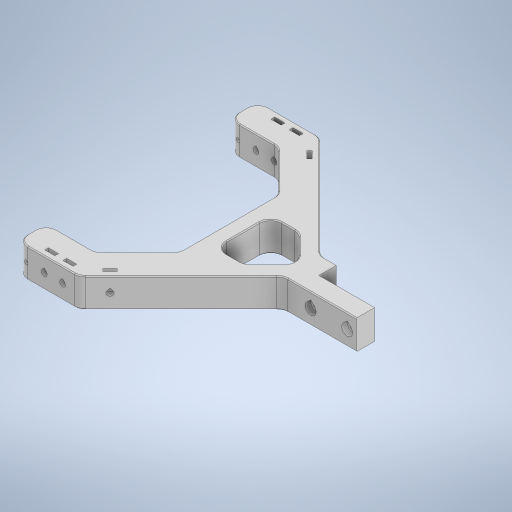
# Autodesk Inventor part: middle_Y
Saved by Autodesk Inventor 2023.1 (Build 271208000, 208)
## iProperties
Created: 2023-11-20
Part Number: middle_Y
Material: Všeobecné
Document SubType Name: Modeling
Designer: zavrel
Density: 1 g/cm^3
Appearance: Výchozí
Author: zavrel
Autodesk Inventor part; units mm, degrees
ref_plane "YZ Plane" through (0, 0, 0) normal (1, 0, 0) x (0, 1, 0)
ref_plane "XZ Plane" through (0, 0, 0) normal (0, 1, 0) x (-1, 0, 0)
ref_plane "XY Plane" through (0, 0, 0) normal (0, 0, 1) x (1, 0, 0)
sketch "Náčrt1" plane through (0, 0, 0) normal (0, 1, 0) x (-1, 0, 0)
  line L0 (0, 0) -> (0, 10)
  line L1 (0, 10) -> (40, 10)
  line L2 (40, 10) -> (96, 66)
  line L3 (96, 66) -> (130, 66)
  line L4 (130, 66) -> (130, 50)
  line L5 (130, 50) -> (102.627417, 50)
  line L6 (102.627417, 50) -> (80, 27.372583)
  line L7 (80, 27.372583) -> (80, 0)
  line L8 (0, 0) -> (258.3801, 0) construction
  line L9 (0, 0) -> (0, -10)
  line L10 (0, -10) -> (40, -10)
  line L11 (40, -10) -> (96, -66)
  line L12 (96, -66) -> (130, -66)
  line L13 (130, -66) -> (130, -50)
  line L14 (130, -50) -> (102.627417, -50)
  line L15 (102.627417, -50) -> (80, -27.372583)
  line L16 (80, -27.372583) -> (80, 0)
  dimension "d0" = 16
  dimension "d2" = 16
  dimension "d3" = 45
  dimension "d4" = 10
  dimension "d5" = 40
  dimension "d7" = 100
  dimension "d9" = 80
  dimension "d10" = 50
  constraints: 34 end point, 7 symmetric about line, 3 perpendicular, 2 horizontal, 2 parallel, 1 point on line, 1 vertical
  measures "d0" distance of L3.end L4.end
  measures "d2" distance between parallel lines of L6 L2
  measures "d3" angle of L8 L2
  measures "d4" distance between parallel lines of L8 L1
  measures "d5" distance of L9.end L10.end
  measures "d7" distance between parallel lines of L14 L5
  measures "d9" distance between parallel lines of L9 L16
  measures "d10" distance between parallel lines of L16 L13
extrude "Vysunutí1" add sketch "Náčrt1" along normal blind 16
sketch "Náčrt2" plane through (-96, 0, -66) normal (0, 0, -1) x (-1, 0, 0)
  line L0 (0, 0) -> (34, 0)
  line L1 (34, 0) -> (34, 16)
  line L2 (0, 16) -> (34, 16)
  line L3 (0, 0) -> (0, 16)
  line L4 (34, 8) -> (0, 8) construction
  circle A0 centre (29, 8) radius 1
  circle A1 centre (19, 8) radius 1.6
  circle A2 centre (9, 8) radius 1.6
  line L5 (19, 8) -> (19, 11.827062) construction
  line L6 (19, 10.262742) -> (20.131371, 9.131371)
  line L7 (19, 10.262742) -> (17.868629, 9.131371)
  line L8 (9, 10.262742) -> (10.131371, 9.131371)
  line L9 (9, 10.262742) -> (7.868629, 9.131371)
  point P0 (-96, 0)
  point P1 (7.868629, 9.131371)
  point P2 (10.131371, 9.131371)
  dimension "d13" = 2
  dimension "d14" = 3.2
  dimension "d15" = 5
  dimension "d16" = 10
  dimension "d17" = 10
  dimension "d22" = 90
  dimension "d23" = 90
  constraints: 12 end point, 4 point on line, 3 centre point, 2 midpoint, 2 point on circle, 2 tangent, 1 equal radius, 1 vertical
  measures "d13" diameter of A0
  measures "d14" diameter of A1
  measures "d15" distance from line of L1 A0.centre
  measures "d16" distance of A0.centre L5.start
  measures "d17" distance of L5.start A2.centre
  measures "d22" angle of L7 L6
  measures "d23" angle of L9 L8
extrude "Vysunutí2" cut sketch "Náčrt2" against normal up to surface (132 mm away) contours A0 | A1 | A1 L7 L6 | A2 | A2 L9 L8
sketch "Náčrt3" plane through (-96, 0, -66) normal (0.7071068, 0, -0.7071068) x (-0.7071068, 0, -0.7071068)
  line L0 (-79.195959, 0) -> (0, 0)
  line L1 (0, 0) -> (0, 16)
  line L2 (-79.195959, 16) -> (0, 16)
  line L3 (-79.195959, 0) -> (-79.195959, 16)
  line L4 (0, 8) -> (-20.182521, 8) construction
  circle A0 centre (-12, 8) radius 1.6
  line L5 (-12, 8) -> (-12, 19.241731) construction
  line L6 (-12, 10.262742) -> (-10.868629, 9.131371)
  line L7 (-12, 10.262742) -> (-13.131371, 9.131371)
  point P0 (-114.551299, 0)
  dimension "d20" = 3.2
  dimension "d21" = 90
  dimension "d26" = 12
  constraints: 8 end point, 2 point on circle, 2 point on line, 2 tangent, 1 centre point, 1 horizontal, 1 midpoint, 1 vertical
  measures "d20" diameter of A0
  measures "d21" angle of L7 L6
  measures "d26" distance from line of L1 L5.start
extrude "Vysunutí3" cut sketch "Náčrt3" against normal up to surface (16 mm away) contours A0 | A0 L7 L6
sketch "Náčrt4" plane through (-40, 0, 10) normal (0.7071068, 0, 0.7071068) x (0.7071068, 0, -0.7071068)
  line L0 (-79.195959, 0) -> (0, 0)
  line L1 (0, 0) -> (0, 16)
  line L2 (-79.195959, 16) -> (0, 16)
  line L3 (-79.195959, 0) -> (-79.195959, 16)
  line L4 (-79.195959, 8) -> (0, 8) construction
  circle A0 centre (-67.195959, 8) radius 1.6
  line L5 (-67.195959, 8) -> (-67.195959, 16) construction
  line L6 (-67.195959, 10.262742) -> (-68.32733, 9.131371)
  line L7 (-67.195959, 10.262742) -> (-66.064589, 9.131371)
  point P0 (35.355339, 0)
  dimension "d27" = 3.2
  dimension "d28" = 12
  dimension "d29" = 90
  constraints: 8 end point, 3 point on line, 2 midpoint, 2 point on circle, 2 tangent, 1 centre point, 1 perpendicular
  measures "d27" diameter of A0
  measures "d28" distance from line of L3 L5.start
  measures "d29" angle of L7 L6
extrude "Vysunutí4" cut sketch "Náčrt4" against normal up to surface (16 mm away) contours A0 | A0 L6 L7
sketch "Sketch6" plane through (0, 16, 0) normal (0, 1, 0) x (1, 0, 0)
  line L0 (-130, -66) -> (-96, -66)
  line L1 (-96, -66) -> (-40, -10)
  line L2 (-96, 66) -> (-130, 66)
  line L3 (-40, 10) -> (-96, 66)
  line L4 (-117.75, -63) -> (-112.25, -63)
  line L5 (-112.25, -63) -> (-112.25, -61)
  line L6 (-112.25, -61) -> (-117.75, -61)
  line L7 (-117.75, -61) -> (-117.75, -63)
  line L8 (-117.75, -63) -> (-112.25, -61) construction
  line L9 (-112.25, -63) -> (-117.75, -61) construction
  line L10 (-107.75, -63) -> (-102.25, -63)
  line L11 (-102.25, -63) -> (-102.25, -61)
  line L12 (-102.25, -61) -> (-107.75, -61)
  line L13 (-107.75, -61) -> (-107.75, -63)
  line L14 (-107.75, -63) -> (-102.25, -61) construction
  line L15 (-102.25, -63) -> (-107.75, -61) construction
  line L16 (-87.691495, -53.448855) -> (-91.580583, -57.337942)
  line L17 (-91.580583, -57.337942) -> (-92.994796, -55.923728)
  line L18 (-92.994796, -55.923728) -> (-89.105709, -52.034641)
  line L19 (-89.105709, -52.034641) -> (-87.691495, -53.448855)
  line L20 (-87.691495, -53.448855) -> (-92.994796, -55.923728) construction
  line L21 (-91.580583, -57.337942) -> (-89.105709, -52.034641) construction
  line L22 (-130, -50) -> (-130, -66)
  line L23 (-96, -66) -> (-99.792003, -62.207997) construction
  line L24 (-80, 27.372583) -> (-80, -27.372583)
  line L25 (-80, 0) -> (-94.372603, 0) construction
  line L26 (-117.75, 63) -> (-112.25, 63)
  line L27 (-112.25, 63) -> (-112.25, 61)
  line L28 (-112.25, 61) -> (-117.75, 61)
  line L29 (-117.75, 61) -> (-117.75, 63)
  line L30 (-117.75, 63) -> (-112.25, 61) construction
  line L31 (-112.25, 63) -> (-117.75, 61) construction
  line L32 (-107.75, 63) -> (-102.25, 63)
  line L33 (-102.25, 63) -> (-102.25, 61)
  line L34 (-102.25, 61) -> (-107.75, 61)
  line L35 (-107.75, 61) -> (-107.75, 63)
  line L36 (-107.75, 63) -> (-102.25, 61) construction
  line L37 (-102.25, 63) -> (-107.75, 61) construction
  line L38 (-87.691495, 53.448855) -> (-91.580583, 57.337942)
  line L39 (-91.580583, 57.337942) -> (-92.994796, 55.923728)
  line L40 (-92.994796, 55.923728) -> (-89.105709, 52.034641)
  line L41 (-89.105709, 52.034641) -> (-87.691495, 53.448855)
  line L42 (-87.691495, 53.448855) -> (-92.994796, 55.923728) construction
  line L43 (-91.580583, 57.337942) -> (-89.105709, 52.034641) construction
  point P0 (0, 0)
  point P1 (-115, -62)
  point P2 (-105, -62)
  point P3 (-90.343146, -54.686292)
  point P4 (-115, 62)
  point P5 (-105, 62)
  point P6 (-90.343146, 54.686292)
  dimension "d53" = 2
  dimension "d54" = 5.5
  dimension "d55" = 15
  dimension "d56" = 10
  dimension "d57" = 12
  dimension "d60" = 3
  dimension "d61" = 3
  constraints: 76 end point, 15 symmetric about line, 9 midpoint, 8 parallel, 4 equal length, 3 horizontal, 3 perpendicular, 2 point on line
  measures "d53" distance of L6.end L4.start
  measures "d54" distance of L5.end L6.end
  measures "d55" distance from line of L22 point (-115, -62)
  measures "d56" distance of point (-105, -62) point (-115, -62)
  measures "d57" distance from line of point (-90.343, -54.686) L23
  measures "d60" distance between parallel lines of L1 L16
  measures "d61" distance between parallel lines of L0 L10
extrude "Extrusion5" cut sketch "Sketch6" against normal blind 11
sketch "Sketch7" plane through (0, 0, -10) normal (0, 0, -1) x (-1, 0, 0)
  line L0 (0, 0) -> (40, 0)
  line L1 (40, 0) -> (40, 16)
  line L2 (0, 16) -> (40, 16)
  line L3 (0, 0) -> (0, 16)
  line L4 (0, 8) -> (40, 8) construction
  line L5 (40, 0) -> (40, 16) construction
  circle A0 centre (5, 8) radius 1.6
  circle A1 centre (25, 8) radius 1.6
  line L6 (5, 8) -> (5, 13.898032) construction
  line L7 (5, 10.262742) -> (3.868629, 9.131371)
  line L8 (5, 10.262742) -> (6.131371, 9.131371)
  line L9 (25, 10.262742) -> (23.868629, 9.131371)
  line L10 (25, 10.262742) -> (26.131371, 9.131371)
  dimension "d62" = 3.2
  dimension "d63" = 5
  dimension "d64" = 20
  dimension "d65" = 90
  dimension "d66" = 90
  constraints: 12 end point, 3 point on line, 1 centre point, 1 midpoint, 1 vertical, 7 other
  measures "d63" distance from line of L3 L6.start
  measures "d64" distance of A1.centre L6.start
  measures "d65" angle of L8 L7
  measures "d66" angle of L10 L9
extrude "Extrusion6" cut sketch "Sketch7" against normal through all contours A0 | A0 L7 L8 | A1 | A1 L9 L10
sketch "Sketch8" plane through (0, 0, -10) normal (0, 0, -1) x (-1, 0, 0)
  line L0 (23.868629, 9.131371) -> (25, 10.262742)
  line L1 (25, 10.262742) -> (26.131371, 9.131371)
  arc A0 (23.868629, 9.131371) -> (26.131371, 9.131371) centre (25, 8) ccw
  line L2 (3.868629, 9.131371) -> (5, 10.262742)
  line L3 (5, 10.262742) -> (6.131371, 9.131371)
  arc A1 (3.868629, 9.131371) -> (6.131371, 9.131371) centre (5, 8) ccw
  line L4 (0, 0) -> (40, 0)
  line L5 (40, 0) -> (40, 16)
  line L6 (0, 16) -> (40, 16)
  line L7 (0, 0) -> (0, 16)
  line L8 (40, 16) -> (0, 16)
  line L9 (30.5, 16) -> (30.5, 0)
  line L10 (0, 0) -> (40, 0)
  dimension "d69" = 30.5
  constraints: 2 end point, 2 point on line, 1 perpendicular
  measures "d69" distance between parallel lines of L9 L7
extrude "Extrusion7" cut sketch "Sketch8" against normal blind 10 contours L7 L6 L9 L4
sketch "Sketch9" plane through (0, 16, 0) normal (0, 1, 0) x (1, 0, 0)
  line L0 (-80, 27.372583) -> (-80, -27.372583) construction
  line L1 (-80, 0) -> (-30.631309, 0) construction
  line L2 (-72, 0) -> (-72, -15)
  line L3 (-72, -15) -> (-56.313708, -15)
  line L4 (-56.313708, -15) -> (-41.313708, 0)
  line L5 (0, 0) -> (-30.5, 0)
  line L6 (-30.5, 0) -> (-30.5, 10)
  line L7 (-30.5, 10) -> (-40, 10)
  line L8 (-40, 10) -> (-96, 66)
  line L9 (-96, 66) -> (-130, 66)
  line L10 (-130, 66) -> (-130, 50)
  line L11 (-130, 50) -> (-102.627417, 50)
  line L12 (-102.627417, 50) -> (-80, 27.372583)
  line L13 (-80, 27.372583) -> (-80, -27.372583)
  line L14 (-80, -27.372583) -> (-102.627417, -50)
  line L15 (-102.627417, -50) -> (-130, -50)
  line L16 (-130, -50) -> (-130, -66)
  line L17 (-130, -66) -> (-96, -66)
  line L18 (-96, -66) -> (-40, -10)
  line L19 (-40, -10) -> (0, -10)
  line L20 (0, -10) -> (0, 0)
  line L21 (-112.25, 63) -> (-112.25, 61)
  line L22 (-112.25, 61) -> (-117.75, 61)
  line L23 (-117.75, 61) -> (-117.75, 63)
  line L24 (-117.75, 63) -> (-112.25, 63)
  line L25 (-107.75, -61) -> (-102.25, -61)
  line L26 (-102.25, -61) -> (-102.25, -63)
  line L27 (-102.25, -63) -> (-107.75, -63)
  line L28 (-107.75, -63) -> (-107.75, -61)
  line L29 (-117.75, -61) -> (-112.25, -61)
  line L30 (-112.25, -61) -> (-112.25, -63)
  line L31 (-112.25, -63) -> (-117.75, -63)
  line L32 (-117.75, -63) -> (-117.75, -61)
  line L33 (-107.75, 61) -> (-107.75, 63)
  line L34 (-107.75, 63) -> (-102.25, 63)
  line L35 (-102.25, 63) -> (-102.25, 61)
  line L36 (-102.25, 61) -> (-107.75, 61)
  line L37 (-91.580583, -57.337942) -> (-92.994796, -55.923728)
  line L38 (-92.994796, -55.923728) -> (-89.105709, -52.034641)
  line L39 (-89.105709, -52.034641) -> (-87.691495, -53.448855)
  line L40 (-87.691495, -53.448855) -> (-91.580583, -57.337942)
  line L41 (-87.691495, 53.448855) -> (-89.105709, 52.034641)
  line L42 (-89.105709, 52.034641) -> (-92.994796, 55.923728)
  line L43 (-92.994796, 55.923728) -> (-91.580583, 57.337942)
  line L44 (-91.580583, 57.337942) -> (-87.691495, 53.448855)
  line L45 (-72, 0) -> (-72, 15)
  line L46 (-72, 15) -> (-56.313708, 15)
  line L47 (-56.313708, 15) -> (-41.313708, 0)
  line L48 (-96, -66) -> (-40, -10)
  dimension "d72" = 30
  dimension "d73" = 8
  dimension "d74" = 8
  constraints: 14 end point, 2 point on line, 2 symmetric about line, 1 horizontal, 1 midpoint, 1 parallel, 1 perpendicular, 1 vertical
  measures "d72" distance between parallel lines of L46 L3
  measures "d73" distance between parallel lines of L0 L2
  measures "d74" distance between parallel lines of L18 L4
extrude "Extrusion8" cut sketch "Sketch9" against normal through all contours L45 L46 L47 L4 L3 L2
sketch "Sketch10" plane through (-40, 0, 10) normal (0, 0, 1) x (1, 0, 0)
  line L0 (15, 10.262742) -> (16.131371, 9.131371)
  arc A0 (13.868629, 9.131371) -> (16.131371, 9.131371) centre (15, 8) ccw
  line L1 (13.868629, 9.131371) -> (15, 10.262742)
  line L2 (35, 10.262742) -> (36.131371, 9.131371)
  arc A1 (33.868629, 9.131371) -> (36.131371, 9.131371) centre (35, 8) ccw
  line L3 (33.868629, 9.131371) -> (35, 10.262742)
  line L4 (0, 0) -> (40, 0)
  line L5 (40, 0) -> (40, 16)
  line L6 (0, 16) -> (40, 16)
  line L7 (0, 0) -> (0, 16)
  arc A2 (13.868629, 9.131371) -> (16.131371, 9.131371) centre (15, 8) ccw
  circle A3 centre (15, 8) radius 3
  circle A4 centre (35, 8) radius 3
  line L8 (15, 12.242641) -> (12.87868, 10.12132)
  line L9 (15, 12.242641) -> (17.12132, 10.12132)
  line L10 (35, 12.242641) -> (32.87868, 10.12132)
  line L11 (35, 12.242641) -> (37.12132, 10.12132)
  dimension "d77" = 6
  dimension "d78" = 6
  dimension "d79" = 90
  dimension "d80" = 90
  constraints: 8 end point, 2 centre point, 2 coincident, 2 point on circle, 2 tangent, 1 parallel
  measures "d77" diameter of A3
  measures "d78" diameter of A4
  measures "d79" angle of L9 L8
  measures "d80" angle of L11 L10
extrude "Extrusion9" cut sketch "Sketch10" against normal blind 3 contours A3 | A3 L8 L9 | A4 | A4 L10 L11
fillet "Fillet1" radius 6 17 edges at (-40, 8, 10) (-40, 8, -10) (-56.3137, 8, 15) (-72, 8, 15) (-41.3137, 8, 0) (-72, 8, -15) (-56.3137, 8, -15) (-80, 8, -27.3726) (-80, 8, 27.3726) (-130, 8, -66) (-130, 8, -50) (-130, 8, 50) (-130, 8, 66) (-102.6274, 8, 50) (-102.6274, 8, -50) (-96, 8, 66) (-96, 8, -66)
chamfer "Chamfer1" distance 0.5 angle 45 59 edges at (-68, 16, 38) (-96.1892, 16, 65.5433) (-18.7574, 16, 10) (-111.2426, 16, 66) (-128.2426, 16, 64.2426) (-130, 16, 58) (-128.2426, 16, 51.7574) (-114.5563, 16, 50) (-91.3137, 16, 38.6863) (-128.2426, 16, -51.7574) (-128.2426, 16, -64.2426) (-96.1892, 16, -65.5433) (-70.2426, 16, 13.2426) (-70.2426, 16, -13.2426) (-56.5029, 16, 14.5433) (-56.5029, 16, -14.5433) (-43.799, 16, 0) (-80, 16, 0) (-91.3137, 16, -38.6863) (-114.5563, 16, -50) (-130, 16, -58) (-111.2426, 16, -66) (-68, 16, -38) (-34.0074, 16, -10) (-30.5, 8, -10) (-68, 0, -38) (-96.1892, 0, -65.5433) (-111.2426, 0, -66) (-128.2426, 0, -64.2426) (-130, 0, -58) (-128.2426, 0, -51.7574) (-114.5563, 0, -50) (-91.3137, 0, -38.6863) (-96.1892, 0, 65.5433) (-128.2426, 0, 64.2426) (-128.2426, 0, 51.7574) (-70.2426, 0, -13.2426) (-70.2426, 0, 13.2426) (-56.5029, 0, -14.5433) (-56.5029, 0, 14.5433) (-43.799, 0, 0) (-80, 0, 0) (-91.3137, 0, 38.6863) (-114.5563, 0, 50) (-130, 0, 58) (-111.2426, 0, 66) (-68, 0, 38) (-18.7574, 0, 10) (-34.0074, 0, -10) (-50.0563, 0, 8.7426) (-62.3995, 0, 15) (-72, 0, 0) (-62.3995, 0, -15) (-50.0563, 0, -8.7426) (-50.0563, 16, 8.7426) (-62.3995, 16, 15) (-72, 16, 0) (-62.3995, 16, -15) (-50.0563, 16, -8.7426)
